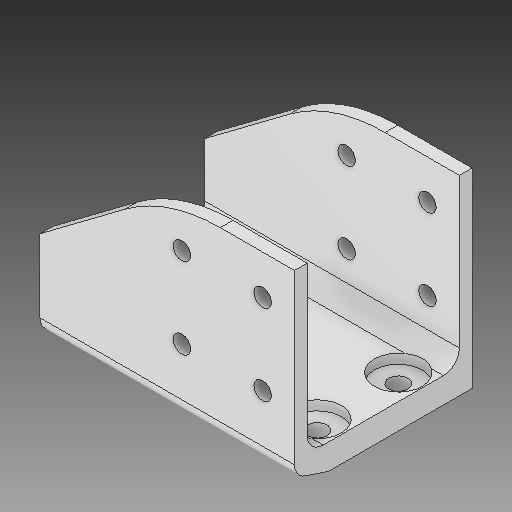
# Autodesk Inventor part: Motor Bracket
Saved by Autodesk Inventor 2019.4 (Build 234330000, 330)
## iProperties
Created: 2020-04-13
Part Number: Motor Bracket
Material: ABS Plastic
Document SubType Name: Modeling
Designer: admin
Density: 1.06 g/cm^3
Appearance: Smooth - White
Author: admin
Autodesk Inventor part; units mm, degrees
ref_plane "YZ Plane" through (0, 0, 0) normal (1, 0, 0) x (0, 1, 0)
ref_plane "XZ Plane" through (0, 0, 0) normal (0, 1, 0) x (-1, 0, 0)
ref_plane "XY Plane" through (0, 0, 0) normal (0, 0, 1) x (1, 0, 0)
sketch "Sketch1" plane through (0, 0, 0) normal (0, 0, 1) x (1, 0, 0)
  line L0 (0, 0) -> (-25.4, 0) construction
  line L1 (-25.4, 0) -> (-25.4, -25.4) construction
  line L2 (-25.4, -25.4) -> (0, -25.4) construction
  line L3 (0, -25.4) -> (0, 0) construction
  circle A0 centre (-25.4, 0) radius 2.75
  circle A1 centre (0, 0) radius 2.75
  circle A2 centre (0, -25.4) radius 2.75
  circle A3 centre (-25.4, -25.4) radius 2.75
  line L4 (-70, 12.3) -> (10, 12.3)
  line L5 (10, 12.3) -> (10, -47.7)
  line L6 (10, -47.7) -> (-70, -47.7)
  line L7 (-70, -47.7) -> (-70, 12.3)
  line L8 (0, -12.7) -> (49.5609, -12.7) construction
  dimension "d0" = 25.4
  dimension "d1" = 25.4
  dimension "d2" = 5.5
  dimension "d3" = 5.5
  dimension "d4" = 5.5
  dimension "d5" = 5.5
  dimension "d6" = 80
  dimension "d8" = 35
  dimension "d9" = 60
  dimension "d10" = 10
  constraints: 19 end point, 4 centre point, 4 coincident, 4 perpendicular, 3 horizontal, 2 parallel, 1 midpoint
  measures "d0" distance of L2.end L0.start
  measures "d1" distance of L1.end L2.end
  measures "d2" diameter of A0
  measures "d3" diameter of A1
  measures "d4" diameter of A2
  measures "d5" diameter of A3
  measures "d6" distance of L4.start L4.end
  measures "d8" distance between parallel lines of L6 L8
  measures "d9" distance of L4.end L5.end
  measures "d10" distance between parallel lines of L5 L3
extrude "Extrusion1" add sketch "Sketch1" along normal blind 4
sketch "Sketch2" plane through (0, 0, 0) normal (0, 0, -1) x (-1, 0, 0)
  line L0 (-10, -39.7) -> (70, -39.7)
  line L1 (-10, -47.7) -> (-10, 12.3) projected
  line L2 (70, -47.7) -> (-10, -47.7) projected
  line L3 (70, 12.3) -> (70, -47.7) projected
  line L4 (-15.5754, -36.9) -> (45.7516, -36.9) construction
  circle A0 centre (25.4, -25.4) radius 2.75 projected
  point P0 (0, 0)
  dimension "d13" = 8
  dimension "d14" = 11.5
  constraints: 4 end point, 2 horizontal, 2 point on line
  measures "d13" distance between parallel lines of L2 L0
  measures "d14" distance from line of A0.centre L4
extrude "Extrusion2" add sketch "Sketch2" along normal blind 47.8 contours L0 L3 L2 L1
sketch "Sketch3" plane through (0, 0, -47.8) normal (0, 0, -1) x (-1, 0, 0)
  circle A0 centre (25.4, -25.4) radius 2.75 projected
  circle A1 centre (0, -25.4) radius 2.75 projected
  circle A2 centre (0, 0) radius 2.75 projected
  circle A3 centre (25.4, 0) radius 2.75 projected
  line L0 (-10, 12.3) -> (70, 12.3) projected
  line L1 (70, 12.3) -> (70, -47.7) projected
  line L2 (70, -47.7) -> (-10, -47.7) projected
  line L3 (-10, -47.7) -> (-10, 12.3) projected
extrude "Extrusion3" add sketch "Sketch3" along normal blind 4
sketch "Sketch4" plane through (-70, -47.7, 4) normal (0, -1, 0) x (1, 0, 0)
  circle A0 centre (72.1064, -15.1125) radius 3 projected
  circle A1 centre (27.275, -15.1125) radius 3 projected
  circle A2 centre (27.275, -40.5125) radius 3 projected
  circle A3 centre (72.1064, -40.5125) radius 3 projected
  point P0 (70, -4)
extrude "Extrusion4" cut sketch "Sketch4" against normal through all
sketch "Sketch5" plane through (-70, -39.7, 0) normal (0, 1, 0) x (1, 0, 0)
  circle A0 centre (27.275, 11.1125) radius 3 projected
  circle A1 centre (27.275, 36.5125) radius 3 projected
  circle A2 centre (72.1064, 11.1125) radius 3 projected
  circle A3 centre (72.1064, 36.5125) radius 3 projected
  point P0 (70, 0)
  constraints: 4 coincident
hole "Hole1" at (-42.725, -39.7, -11.1125) at (-42.725, -39.7, -36.5125) at (2.1064, -39.7, -11.1125) at (2.1064, -39.7, -36.5125) direction (0, -1, 0) diameter 15 depth 3
sketch "Sketch6" plane through (0, 0, 4) normal (0, 0, 1) x (1, 0, 0)
  line L0 (-70, 12.3) -> (-70, -47.7) projected
  line L1 (-70, -17.7) -> (-30, 12.3)
  line L2 (10, 12.3) -> (-70, 12.3) projected
  point P0 (0, 0)
  dimension "d28" = 40
  dimension "d29" = 30
  constraints: 2 end point, 2 midpoint
  measures "d28" horizontal distance of L1.start L1.end
  measures "d29" vertical distance of L1.start L1.end
extrude "Extrusion5" cut sketch "Sketch6" against normal through all
sketch "Sketch7" plane through (10, -47.7, 4) normal (1, 0, 0) x (0, 0, -1)
  line L0 (55.8, 0) -> (0, 0) projected
  line L1 (10.705, 0) -> (0, 3.5)
  line L2 (0, 0) -> (0, 60) projected
  point P0 (4, 47.7)
  dimension "d32" = 10.705
  dimension "d33" = 3.5
  constraints: 2 end point, 2 point on line
  measures "d32" distance of L0.end L1.start
  measures "d33" vertical distance of L1.start L1.end
extrude "Extrusion6" cut sketch "Sketch7" against normal through all
fillet "Fillet1" radius 5 4 edges at (-30, -44.2, 4) (-30, -47.7, -6.705) (-30, -39.7, 0) (-30, -39.7, -47.8)
fillet "Fillet2" radius 50 2 edges at (-30, 12.3, -49.8) (-30, 12.3, 2)
body "Solid1"
